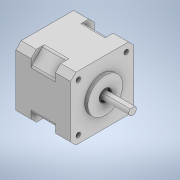
# Autodesk Inventor part: Steppermotor
Saved by Autodesk Inventor 2021 (Build 250183000, 183)
## iProperties
Created: 2021-01-04
Part Number: Steppermotor
Material: Generisch
Document SubType Name: Modeling
Designer: Ctroi
Density: 1 g/cm^3
Appearance: Vorgabe
Author: Ctroi
Autodesk Inventor part; units mm, degrees
ref_plane "YZ Plane" through (0, 0, 0) normal (1, 0, 0) x (0, 1, 0)
ref_plane "XZ Plane" through (0, 0, 0) normal (0, 1, 0) x (-1, 0, 0)
ref_plane "XY Plane" through (0, 0, 0) normal (0, 0, 1) x (1, 0, 0)
sketch "Skizze2" plane through (0, 0, 0) normal (1, 0, 0) x (0, 1, 0)
  line L0 (20.75, -20.75) -> (-20.75, -20.75)
  line L1 (-20.75, -20.75) -> (-20.75, 20.75)
  line L2 (-20.75, 20.75) -> (20.75, 20.75)
  line L3 (20.75, 20.75) -> (20.75, -20.75)
  line L4 (-29.05, 0) -> (29.05, 0) projected
  line L5 (0, -29.05) -> (0, 29.05) projected
  point P0 (0, 0)
  dimension "d0" = 41.5
  dimension "d1" = 41.5
  constraints: 8 end point, 2 parallel, 1 horizontal, 1 perpendicular, 2 other
  measures "d0" distance of L2.end L1.end
  measures "d1" distance of L1.end L0.end
extrude "Extrusion1" add sketch "Skizze2" along normal blind 10
chamfer "Fase1" distance 3.5 angle 45 4 edges at (5, 20.75, 20.75) (5, 20.75, -20.75) (5, -20.75, -20.75) (5, -20.75, 20.75)
sketch "Skizze5" plane through (10, 0, 0) normal (1, 0, 0) x (0, 0, -1)
  line L0 (20.75, 20.75) -> (-20.75, 20.75)
  line L1 (-20.75, 20.75) -> (-20.75, -20.75)
  line L2 (-20.75, -20.75) -> (20.75, -20.75)
  line L3 (20.75, -20.75) -> (20.75, 20.75)
  line L4 (0, -29.064) -> (0, 29.1338) projected
  line L5 (17.25, 20.75) -> (-17.25, 20.75) projected
  line L6 (29.05, 0) -> (-29.05, 0) projected
  line L7 (20.75, -17.25) -> (20.75, 17.25) projected
  line L8 (20.75, 12.75) -> (12.75, 20.75)
  line L9 (17.25, 20.75) -> (20.75, 17.25) projected
  line L10 (-12.75, 20.75) -> (-20.75, 12.75)
  line L11 (-20.75, -12.75) -> (-12.75, -20.75)
  line L12 (12.75, -20.75) -> (20.75, -12.75)
  point P0 (0, 0)
  dimension "d11" = 41.5
  dimension "d12" = 41.5
  dimension "d20" = 8
  dimension "d21" = 8
  dimension "d24" = 360
  constraints: 16 end point, 2 parallel, 2 point on line, 1 horizontal, 1 perpendicular, 15 other
  measures "d11" distance of L2.end L1.end
  measures "d12" distance of L1.end L0.end
  measures "d20" distance of L0.start L8.start
  measures "d21" distance from line of L3 L8.end
extrude "Extrusion5" add sketch "Skizze5" along normal blind 16 contours L8 L3 L6 L4 L0 | L4 L6 L1 L10 L0 | L3 L12 L2 L4 L6 | L4 L2 L11 L1 L6
sketch "Skizze6" plane through (26, 0, 0) normal (1, 0, 0) x (0, 0, -1)
  line L0 (20.75, 20.75) -> (-20.75, 20.75)
  line L1 (-20.75, 20.75) -> (-20.75, -20.75)
  line L2 (-20.75, -20.75) -> (20.75, -20.75)
  line L3 (20.75, -20.75) -> (20.75, 20.75)
  line L4 (29.05, 0) -> (-29.05, 0) projected
  line L5 (0, -29.05) -> (0, 29.05) projected
  line L6 (20.75, 12.75) -> (20.75, 17.25) projected
  line L7 (20.75, 17.25) -> (17.25, 20.75)
  line L8 (-17.25, 20.75) -> (-20.75, 17.25)
  line L9 (-20.75, -17.25) -> (-17.25, -20.75)
  line L10 (17.25, -20.75) -> (20.75, -17.25)
  point P0 (0, 0)
  dimension "d28" = 41.5
  dimension "d29" = 41.5
  dimension "d32" = 360
  constraints: 16 end point, 2 parallel, 1 horizontal, 1 perpendicular, 15 other
  measures "d28" distance of L2.end L1.end
  measures "d29" distance of L1.end L0.end
extrude "Extrusion6" add sketch "Skizze6" along normal blind 10 contours L7 L3 L4 L5 L0 | L5 L4 L1 L8 L0 | L5 L2 L9 L1 L4 | L4 L3 L10 L2 L5
fillet "Rundung1" radius 2 8 edges at (18, 12.75, -20.75) (18, 20.75, -12.75) (18, -12.75, -20.75) (18, -20.75, -12.75) (18, -20.75, 12.75) (18, -12.75, 20.75) (18, 12.75, 20.75) (18, 20.75, 12.75)
sketch "Skizze7" plane through (36, 0, 0) normal (1, 0, 0) x (0, 0, -1)
  circle A0 centre (0, 0) radius 11.5
  circle A1 centre (15.75, -15.75) radius 1.5
  circle A2 centre (15.75, 15.75) radius 1.5
  circle A3 centre (-15.75, -15.75) radius 1.5
  circle A4 centre (-15.75, 15.75) radius 1.5
  dimension "d37" = 23
  dimension "d61" = 3
  dimension "d62" = 3
  dimension "d67" = 15.75
  dimension "d68" = 15.75
  dimension "d69" = 3
  dimension "d70" = 3
  dimension "d71" = 15.75
  dimension "d72" = 15.75
  constraints: 5 centre point, 1 coincident
  measures "d37" diameter of A0
  measures "d61" diameter of A1
  measures "d62" diameter of A2
  measures "d67" horizontal distance of point (0, 0) A2.centre
  measures "d68" horizontal distance of point (0, 0) A1.centre
  measures "d69" diameter of A3
  measures "d70" diameter of A4
  measures "d71" horizontal distance of point (0, 0) A4.centre
  measures "d72" horizontal distance of point (0, 0) A3.centre
extrude "Extrusion7" add sketch "Skizze7" along normal blind 2 contours A0
sketch "Skizze8" plane through (38, 0, 0) normal (1, 0, 0) x (0, 0, -1)
  circle A0 centre (0, 0) radius 4
  dimension "d40" = 8
  constraints: 1 centre point, 1 coincident
  measures "d40" diameter of A0
extrude "Extrusion8" cut sketch "Skizze8" against normal blind 2
sketch "Skizze9" plane through (36, 0, 0) normal (1, 0, 0) x (0, 0, -1)
  circle A0 centre (0, 0) radius 2.5
  line L0 (2.5, 0) -> (-2.5, 0)
  line L1 (-2.5, 0) -> (-2.5, 2.5)
  line L2 (-2.5, 2.5) -> (2.5, 2.5)
  line L3 (2.5, 2.5) -> (2.5, 0)
  line L4 (2.5, 2.5) -> (-2.5, 2.5)
  line L5 (-2.5, 2.5) -> (-2.5, 2)
  line L6 (-2.5, 2) -> (2.5, 2)
  line L7 (2.5, 2) -> (2.5, 2.5)
  point P0 (1.5, 2)
  point P1 (-1.5, 2)
  dimension "d43" = 5
  dimension "d44" = 0.5
  dimension "d47" = 2
  constraints: 16 end point, 4 parallel, 2 horizontal, 2 perpendicular, 1 coincident, 1 point on line, 3 other
  measures "d44" distance of L5.end L4.end
  measures "d47" distance between parallel lines of L6 L0
extrude "Extrusion9" add sketch "Skizze9" along normal blind 20 contours L0 A0 | A0 L6 L0
sketch "Skizze10" plane through (0, -20.75, -17.25) normal (0, -1, 0) x (1, 0, 0)
  line L0 (0, 0) -> (0, 34.5) projected
  line L1 (0, 24.75) -> (10, 24.75)
  line L2 (10, 24.75) -> (10, 9.75)
  line L3 (10, 9.75) -> (0, 9.75)
  line L4 (0, 9.75) -> (0, 24.75)
  line L5 (0, 17.25) -> (36, 17.25)
  line L6 (36, 34.5) -> (36, 0) projected
  dimension "d48" = 10
  dimension "d49" = 15
  constraints: 10 end point, 2 parallel, 1 horizontal, 1 midpoint, 1 perpendicular, 1 point on line, 1 other
  measures "d48" distance of L2.end L3.end
  measures "d49" distance of L1.end L2.end
extrude "Extrusion10" add sketch "Skizze10" along normal blind 4
extrude "Extrusion11" cut sketch "Skizze7" against normal blind 8 contours A1 | A2 | A3 | A4
